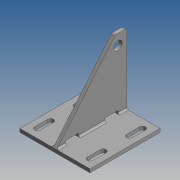
# Autodesk Inventor part: P045_SupportUniversel
Saved by Autodesk Inventor 2021.3 (Build 253353000, 353)
## iProperties
Created: 2022-01-08
Part Number: P045_SupportUniversel
Material: Générique
Document SubType Name: Modeling
Designer: gabri
Density: 1 g/cm^3
Appearance: Par défaut
Author: gabri
Autodesk Inventor part; units mm, degrees
ref_plane "YZ Plane" through (0, 0, 0) normal (1, 0, 0) x (0, 1, 0)
ref_plane "XZ Plane" through (0, 0, 0) normal (0, 1, 0) x (-1, 0, 0)
ref_plane "XY Plane" through (0, 0, 0) normal (0, 0, 1) x (1, 0, 0)
sketch "Sketch2" plane through (0, 0, 0) normal (0, 0, 1) x (1, 0, 0)
  line L0 (40, -40) -> (-40, -40)
  line L1 (-40, -40) -> (-40, 40)
  line L2 (-40, 40) -> (40, 40)
  line L3 (40, 40) -> (40, -40)
  line L4 (-56, 0) -> (56, 0) construction
  line L5 (0, 56) -> (0, -56) construction
  line L6 (-30, 33.25) -> (-30, 11.75) construction
  line L7 (-33.25, 30) -> (-33.25, 15)
  line L8 (-26.75, 15) -> (-26.75, 30)
  arc A0 (-26.75, 30) -> (-33.25, 30) centre (-30, 30) ccw
  arc A1 (-33.25, 15) -> (-26.75, 15) centre (-30, 15) ccw
  line L9 (-26.75, -30) -> (-26.75, -15)
  arc A2 (-26.75, -15) -> (-33.25, -15) centre (-30, -15) ccw
  line L10 (-33.25, -15) -> (-33.25, -30)
  arc A3 (-33.25, -30) -> (-26.75, -30) centre (-30, -30) ccw
  line L11 (33.25, 15) -> (33.25, 30)
  arc A4 (33.25, 30) -> (26.75, 30) centre (30, 30) ccw
  line L12 (26.75, 30) -> (26.75, 15)
  arc A5 (26.75, 15) -> (33.25, 15) centre (30, 15) ccw
  line L13 (33.25, -30) -> (33.25, -15)
  arc A6 (33.25, -15) -> (26.75, -15) centre (30, -15) ccw
  line L14 (26.75, -15) -> (26.75, -30)
  arc A7 (26.75, -30) -> (33.25, -30) centre (30, -30) ccw
  point P0 (0, 0)
  point P1 (0, 0)
  point P2 (0, 0)
  point P3 (-30, 22.5)
  dimension "d10" = 80
  dimension "d11" = 80
  dimension "d12" = 40
  dimension "d13" = 40
  dimension "d14" = 6.5
  dimension "d15" = 10
  dimension "d16" = 10
  dimension "d17" = 15
  dimension "d20" = 45
  dimension "d23" = 60
  dimension "d26" = 6.75
  constraints: 28 end point, 18 point on circle, 8 centre point, 4 tangent, 3 parallel, 2 horizontal, 2 point on line, 2 vertical, 1 coincident, 1 midpoint, 1 perpendicular, 30 other
  measures "d10" distance of L1.end L2.end
  measures "d11" distance of L0.end L1.end
  measures "d12" distance between parallel lines of L4 L2
  measures "d13" distance between parallel lines of L3 L5
  measures "d14" diameter of A1
  measures "d15" distance from line of L1 point (-30, 22.5)
  measures "d16" distance from line of L2 A0.centre
  measures "d17" distance of A1.centre A0.centre
  measures "d20" distance of L8.start L9.start
  measures "d23" distance of L8.start L11.start
  measures "d26" distance between parallel lines of L3 L11
extrude "Extrusion1" add sketch "Sketch2" along normal blind 4
sketch "Sketch3" plane through (0, 0, 0) normal (1, 0, 0) x (0, 1, 0)
  line L0 (33.25, 4) -> (33.25, 0) construction
  line L1 (11.75, 4) -> (11.75, 0) construction
  line L2 (30, 0) -> (15, 0) construction
  line L3 (15, 0) -> (15, 4) construction
  line L4 (30, 4) -> (15, 4) construction
  line L5 (30, 0) -> (30, 4) construction
  line L6 (-15, 0) -> (-30, 0) construction
  line L7 (-30, 0) -> (-30, 4) construction
  line L8 (-15, 4) -> (-30, 4) construction
  line L9 (-15, 0) -> (-15, 4) construction
  line L10 (40, 0) -> (-40, 0) construction
  line L11 (-40, 0) -> (-40, 4) construction
  line L12 (40, 4) -> (-40, 4) construction
  line L13 (40, 0) -> (40, 4) construction
  line L14 (40, 4) -> (40, 84)
  line L15 (40, 84) -> (27.128, 84)
  line L16 (27.128, 84) -> (-40, 4)
  line L17 (-33.25, 4) -> (-33.25, 0) construction
  line L18 (-11.75, 4) -> (-11.75, 0) construction
  line L19 (-30, 8.0014) -> (-15, 8.0014)
  line L20 (15, 8) -> (30, 8)
  line L21 (-15, 8.0014) -> (-15, 4)
  line L22 (-30, 8.0014) -> (-30, 4)
  line L23 (30, 8) -> (30, 4)
  line L24 (15, 8) -> (15, 4)
  line L25 (30, 4) -> (40, 4)
  line L26 (15, 4) -> (-15, 4)
  line L27 (-30, 4) -> (-40, 4)
  point P0 (0, 0)
  dimension "d29" = 80
  dimension "d30" = 4
  dimension "d32" = 130
  dimension "d34" = 4.0014
  constraints: 24 end point, 3 horizontal, 3 perpendicular, 3 vertical, 2 collinear
  measures "d29" distance of L12.start L14.end
  measures "d30" distance between parallel lines of L20 L4
  measures "d32" angle of L15 L16
  measures "d34" distance between parallel lines of L12 L19
extrude "Extrusion2" add sketch "Sketch3" along normal mid plane 4
fillet "Fillet1" radius 2 6 edges at (-2, 0, 4) (-2, 35, 4) (-2, -35, 4) (2, 0, 4) (2, 35, 4) (2, -35, 4)
fillet "Fillet2" radius 2 2 edges at (0, 27.128, 84) (0, 40, 84)
sketch "Sketch4" plane through (2, 0, 0) normal (1, 0, 0) x (0, 0, -1)
  arc A0 (-82, 40) -> (-84, 38) centre (-82, 38) ccw construction
  line L0 (-84, 38) -> (-84, 28.0606) construction
  arc A1 (-84, 28.0606) -> (-83.2856, 26.5285) centre (-82, 28.0606) ccw construction
  line L1 (-83.2856, 26.5285) -> (-6, -38.3218) construction
  line L2 (-6, -30) -> (-6, -38.3218) construction
  line L3 (-6, -30) -> (-8.0014, -30) construction
  line L4 (-8.0014, -30) -> (-8.0014, -15) construction
  line L5 (-8.0014, -15) -> (-6, -15) construction
  line L6 (-6, 15) -> (-6, -15) construction
  line L7 (-6, 15) -> (-8, 15) construction
  line L8 (-8, 15) -> (-8, 30) construction
  line L9 (-8, 30) -> (-6, 30) construction
  line L10 (-6, 40) -> (-6, 30) construction
  line L11 (-6, 40) -> (-82, 40) construction
  point P0 (0, 0)
  point P1 (-72, 30)
  dimension "d39" = 12
  dimension "d40" = 10
  measures "d39" distance from line of point (-72, 30) L0
  measures "d40" distance from line of point (-72, 30) L11
hole "Hole1" at (2, 30, 72) direction (-1, 0, 0) diameter 10 depth 10
equation "\"d41\" = d40"
body "Solid1"
